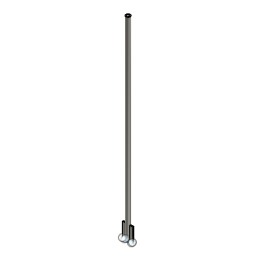
mixer_val v2 (Autodesk Fusion 360 design; units mm, degrees)
Autodesk Fusion 360 part; units mm, degrees
sketch "Sketch1" plane through (0, 0, 0) normal (0, 1, 0) x (1, 0, 0)
  line L0 (0, 0) -> (0, -188.5)
  line L1 (0, 0) -> (-0.6248, 0)
  line L2 (-0.6248, 0) -> (-2.1248, 0)
  line L3 (-2.1248, 0) -> (-2.1248, -188.5)
  line L4 (-2.1248, -188.5) -> (0, -188.5)
  dimension "d1" = 188.5
  dimension "d2" = 1.5
  constraint coincident L0.start L1.start
  constraint vertical L0
  constraint perpendicular L0 L1
  constraint perpendicular L0 L2
  constraint perpendicular L2 L3
  constraint perpendicular L0 L4
  measures "d1" distance of L0.start L0.end
  measures "d2" distance of L1.end L2.end
revolve "Revolve1" add sketch "Sketch1" angle 360 about axis through (0, 0, 0) along (0, 0, 1)
sketch "Sketch2" plane through (0, 0, 0) normal (0, 0, -1) x (1, 0, 0)
  circle A0 centre (0, 0) radius 2.1248
  line L0 (0, 0.5) -> (-3, 0.5)
  line L1 (0, 0.5) -> (3.7205, 0.5)
  line L2 (3.7205, -0.5) -> (-3, -0.5)
  line L3 (0, 0.5) -> (5, 0.5)
  line L4 (5, 0.5) -> (5, -0.5)
  line L5 (5, -0.5) -> (-5, -0.5)
  line L6 (-5, -0.5) -> (-5, 0.5)
  line L7 (-5, 0.5) -> (-5.1, 0.5)
  line L8 (-5, 0.5) -> (5, 0.5)
  dimension "d4" = 0.5
  constraint perpendicular L1 L4
  constraint perpendicular L4 L5
  constraint perpendicular L5 L6
  constraint perpendicular L6 L7
  measures "d4" distance of A0.centre L0.start
extrude "Extrude2" add sketch "Sketch2" against normal blind 14 contours A0 L0 L2 L5 L6 L8
extrude "Extrude1" add sketch "Sketch2" against normal blind 14 contours A0 L1 L2 L3 L4 L5 L8
hole "Hole1" at (0, 0, 188.5) direction (0, 0, -1) diameter 2.529 depth 25 tip angle 118
thread "Thread1" "ISO Metric profile 3.0 M3x0.5 6H"
